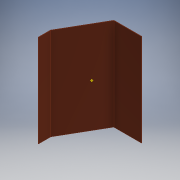
# Autodesk Inventor part: Part1 example centroid
Saved by Autodesk Inventor 2018 (Build 220112000, 112)
## iProperties
Created: 2018-06-12
Part Number: Part1 example centroid
Material: Copper, Wrought
Document SubType Name: Sheet Metal
Designer: P446509
Mass: 41823.5 g
Surface Area: 18906.5 cm^2
Volume: 4678.24 cm^3
Density: 8.94 g/cm^3
Sheet Metal Rule: Default_mm
Appearance: Copper - Satin
Author: P446509
Autodesk Inventor part; units mm, degrees
note: some values were not read from the file. Chosen so that the rebuilt part matches the saved one: flange form of "Plate1".
ref_plane "YZ Plane" through (0, 0, 0) normal (1, 0, 0) x (0, 1, 0)
ref_plane "XZ Plane" through (0, 0, 0) normal (0, 1, 0) x (-1, 0, 0)
ref_plane "XY Plane" through (0, 0, 0) normal (0, 0, 1) x (1, 0, 0)
sketch "Sketch1" plane through (0, 0, 0) normal (0, 0, 1) x (1, 0, 0)
  line L0 (0, 0) -> (-300, 0)
  line L1 (-300, 0) -> (-550, -433.0127)
  line L2 (-550, -433.0127) -> (-550, -565.3325)
  dimension "d0" = 300
  dimension "d1" = 500
  dimension "d2" = 120
  measures "d0" distance of L0.start L0.end
  measures "d1" distance of L0.end L1.end
  measures "d2" angle of L0 L1
contour flange "Contour Flange1" sketch "Sketch1" thickness 5 bend radius 5 width 1000 along (0, 0, 1) mid plane yes both sides no wall seen from (-150, 0, 0) lies toward (0, 1, 0) curves L0 L1 L2
bend "Bend1"
corner "Corner1"
equation "\"d3\" = Thickness"
equation "\"d4\" = BendReliefWidth"
equation "\"d5\" = BendReliefDepth"
equation "\"d6\" = MinimumRemnant"
equation "\"d7\" = TransitionRadius"
equation "\"d9\" = BendRadius"
equation "\"d11\" = CornerReliefSize"
equation "\"d12\" = GapSize"
equation "\"d13\" = JacobiRadiusSize"
equation "\"BendRadius\" = Thickness"
equation "\"BendReliefWidth\" = Thickness"
equation "\"BendReliefDepth\" = 0.5 * Thickness"
equation "\"TransitionRadius\" = BendRadius"
equation "\"JacobiRadiusSize\" = BendRadius"
equation "\"GapSize\" = Thickness"
equation "\"Thickness\" = 5"
equation "\"MinimumRemnant\" = 10"
equation "\"CornerReliefSize\" = 20"
body "Solid1"
